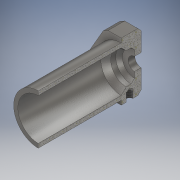
# Autodesk Inventor part: piston_reservoir
Saved by Autodesk Inventor 2019 (Build 230136000, 136)
## iProperties
Created: 2019-03-25
Part Number: piston_reservoir
Material: Acier, galvanisé
Document SubType Name: Modeling
Designer: theor
Density: 7.85 g/cm^3
Appearance: Galvanisé
Mass: 159.268 g
Surface Area: 123.829 cm^2
Volume: 20.289 cm^3
Author: theor
Autodesk Inventor part; units mm, degrees
ref_plane "YZ Plane" through (0, 0, 0) normal (1, 0, 0) x (0, 1, 0)
ref_plane "XZ Plane" through (0, 0, 0) normal (0, 1, 0) x (-1, 0, 0)
ref_plane "XY Plane" through (0, 0, 0) normal (0, 0, 1) x (1, 0, 0)
sketch "Esquisse1" plane through (0, 0, 0) normal (1, 0, 0) x (0, 1, 0)
  line L0 (0, 0) -> (0, 68.1349)
  line L1 (15, 62) -> (15, 12)
  line L2 (15.5, 0) -> (4, 0)
  line L3 (4, 0) -> (4, 4)
  line L4 (4, 4) -> (9.5, 4)
  line L5 (12.5, 12) -> (12.5, 62)
  line L6 (15, 62) -> (12.5, 62)
  line L7 (15, 12) -> (17.5, 12)
  line L8 (17.5, 12) -> (17.5, 2)
  line L9 (17.5, 2) -> (15.5, 0)
  line L10 (12.5, 12) -> (9.5, 9)
  line L11 (9.5, 9) -> (9.5, 4)
  dimension "d0" = 50
  dimension "d1" = 30
  dimension "d2" = 8
  dimension "d3" = 4
  dimension "d4" = 2.5
  dimension "d5" = 2.5
  dimension "d6" = 2
  dimension "d7" = 2
  dimension "d8" = 10
  dimension "d26" = 3
  dimension "d27" = 3
  constraints: 24 end point, 6 vertical, 4 horizontal, 2 horizontal alignment
  measures "d0" distance of L1.start L1.end
  measures "d1" diameter of L1 L0
  measures "d2" diameter of L3 L0
  measures "d3" distance of L2.end L3.end
  measures "d4" distance between parallel lines of L1 L5
  measures "d5" distance of L1.end L7.end
  measures "d6" horizontal distance of L8.end L2.start
  measures "d7" horizontal distance of L8.end L2.start
  measures "d8" distance of L7.end L8.end
  measures "d26" horizontal distance of L5.start L10.end
  measures "d27" horizontal distance of L5.start L10.end
revolve "Révolution1" add sketch "Esquisse1" angle 360 about axis through (0, 0, 0) along (0, 0, 1)
ref_plane "Plan de construction1" through (0, 0, 2) normal (0, 0, -1) x (-1, 0, 0)
sketch "Esquisse3" plane through (0, 0, 2) normal (0, 0, -1) x (-1, 0, 0)
  line L0 (10.1036, 17.5) -> (20.2073, 0)
  line L1 (20.2073, 0) -> (10.1036, -17.5)
  line L2 (10.1036, -17.5) -> (-10.1036, -17.5)
  line L3 (-10.1036, -17.5) -> (-20.2073, 0)
  line L4 (-20.2073, 0) -> (-10.1036, 17.5)
  line L5 (-10.1036, 17.5) -> (10.1036, 17.5)
  circle A0 centre (0, 0) radius 17.5 projected
  constraints: 12 end point, 1 coincident, 1 horizontal, 1 tangent, 13 other
extrude "Extrusion1" add sketch "Esquisse3" against normal blind 10 contours L0 A0 L5 | L0 L1 A0 | A0 L4 L5 | A0 L3 L4 | L1 L2 A0 | A0 L2 L3
chamfer "Chanfrein1" distance 2 angle 45 1 edges at (0, -9.5, 4)
chamfer "Chanfrein2" distance 2 angle 45 6 edges at (10.1036, 17.5, 7) (-10.1036, 17.5, 7) (-20.2073, 0, 7) (-10.1036, -17.5, 7) (10.1036, -17.5, 7) (20.2073, 0, 7)
sketch "Esquisse4" plane through (-8.1036, -17.5, 2) normal (0, -1, 0) x (1, 0, 0)
  line L0 (16.2073, 10) -> (16.2073, 0) projected
  line L1 (0, 10) -> (16.2073, 10) projected
  line L2 (0, 0) -> (0, 10) projected
  line L3 (0, 0) -> (8.1036, 0) projected
  line L4 (8.1036, 0) -> (16.2073, 0) projected
  point P0 (8.1036, -2)
  point P1 (8.1036, 5)
  point P2 (16.2073, 5)
  constraints: 1 horizontal alignment, 1 midpoint, 1 vertical alignment
hole "Perçage1" at (0, -17.5, 7) direction (0, 1, 0) diameter 4.134 depth 5 tip angle 118 thread size "M5x0.8" class "6H" standard "ISO Metric profile"
equation "\"d7\" = d6"
equation "\"d27\" = d26"
